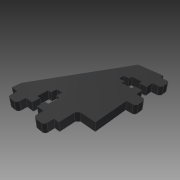
# Autodesk Inventor part: x_motor_cable_mount_brace
Saved by Autodesk Inventor 2014 (Build 180170000, 170)
## iProperties
Created: 2013-12-02
Part Number: x_motor_cable_mount_brace
Material: Generic
Document SubType Name: Modeling
Designer: buben
Density: 1 g/cm^3
Appearance: Anodized - Dark Gray
Author: buben
Subject: Laser Cutted
Autodesk Inventor part; units mm, degrees
ref_plane "YZ Plane" through (0, 0, 0) normal (1, 0, 0) x (0, 1, 0)
ref_plane "XZ Plane" through (0, 0, 0) normal (0, 1, 0) x (-1, 0, 0)
ref_plane "XY Plane" through (0, 0, 0) normal (0, 0, 1) x (1, 0, 0)
sketch "Sketch1" plane through (0, 0, 0) normal (0, 0, 1) x (1, 0, 0)
  line L0 (0, 0) -> (52, 0)
  line L1 (52, 0) -> (52, 68.9)
  line L2 (52, 68.9) -> (34, 68.9)
  line L3 (34, 68.9) -> (0, 6)
  line L4 (0, 6) -> (0, 0)
  dimension "d0" = 52
  dimension "d1" = 6
  dimension "d2" = 18
  dimension "d3" = 68.9
  constraints: 10 end point, 2 parallel, 1 horizontal, 1 perpendicular
  measures "d0" distance of L0.start L0.end
  measures "d1" distance of L3.end L0.start
  measures "d2" distance of L1.end L2.end
  measures "d3" distance of L0.end L1.end
extrude "Extrusion1" add sketch "Sketch1" along normal blind 6
sketch "Sketch2" plane through (0, 0, 6) normal (0, 0, 1) x (1, 0, 0)
  line L0 (0, 0) -> (52, 0) projected
  line L1 (52, 0) -> (52, 68.9) projected
  line L2 (18.75, 16.3) -> (23.25, 16.3)
  line L3 (23.25, 0) -> (18.75, 0)
  line L4 (25.75, 12.3) -> (25.75, 5)
  line L5 (16.25, 5) -> (16.25, 12.3)
  line L6 (39.7, 55.15) -> (47, 55.15)
  line L7 (47, 45.65) -> (39.7, 45.65)
  line L8 (52, 52.65) -> (52, 48.15)
  line L9 (35.7, 48.15) -> (35.7, 52.65)
  line L10 (16.25, 12.3) -> (18.75, 12.3)
  line L11 (23.25, 12.3) -> (25.75, 12.3)
  line L12 (18.75, 0) -> (18.75, 5)
  line L13 (18.75, 12.3) -> (18.75, 16.3)
  line L14 (25.75, 5) -> (23.25, 5)
  line L15 (18.75, 5) -> (16.25, 5)
  line L16 (23.25, 16.3) -> (23.25, 12.3)
  line L17 (23.25, 5) -> (23.25, 0)
  line L18 (52, 48.15) -> (47, 48.15)
  line L19 (39.7, 48.15) -> (35.7, 48.15)
  line L20 (35.7, 52.65) -> (39.7, 52.65)
  line L21 (47, 52.65) -> (52, 52.65)
  line L22 (39.7, 45.65) -> (39.7, 48.15)
  line L23 (39.7, 52.65) -> (39.7, 55.15)
  line L24 (47, 55.15) -> (47, 52.65)
  line L25 (47, 48.15) -> (47, 45.65)
  point P0 (35.7, 50.4)
  point P1 (21, 16.3)
  dimension "d6" = 4.5
  dimension "d7" = 2.5
  dimension "d8" = 2.5
  dimension "d9" = 5
  dimension "d10" = 4
  dimension "d11" = 7.3
  dimension "d12" = 4.5
  dimension "d13" = 2.5
  dimension "d14" = 2.5
  dimension "d15" = 4
  dimension "d16" = 5
  dimension "d17" = 7.3
  dimension "d19" = 31
  dimension "d39" = 18.5
  constraints: 48 end point, 20 parallel, 10 collinear, 8 perpendicular, 6 horizontal, 2 midpoint
  measures "d6" distance of L2.start L2.end
  measures "d7" distance of L11.start L4.start
  measures "d8" distance of L5.end L10.end
  measures "d9" distance of L14.end L3.start
  measures "d10" distance of L2.end L11.start
  measures "d11" distance of L4.start L4.end
  measures "d12" distance of L9.start L9.end
  measures "d13" distance of L20.end L6.start
  measures "d14" distance of L7.end L19.start
  measures "d15" distance of L19.start L9.start
  measures "d16" distance of L8.end L18.end
  measures "d17" distance of L7.start L7.end
  measures "d19" distance from line of L1 point (21, 16.3)
  measures "d39" vertical distance of L1.end point (35.7, 50.4)
extrude "Extrusion2" cut sketch "Sketch2" against normal blind 6
sketch "Sketch3" plane through (0, 0, 6) normal (0, 0, 1) x (1, 0, 0)
  line L0 (23.25, 0) -> (52, 0) projected
  line L1 (52, 0) -> (52, 48.15) projected
  line L2 (35.7, 48.15) -> (35.7, 52.65) projected
  line L3 (52, 52.65) -> (52, 68.9) projected
  line L4 (0, 0) -> (18.75, 0) projected
  line L5 (18.75, 16.3) -> (23.25, 16.3) projected
  line L6 (5.5, 0) -> (13.5, 0)
  line L7 (13.5, 0) -> (13.5, -4)
  line L8 (11.5, -6) -> (7.5, -6)
  line L9 (5.5, -4) -> (5.5, 0)
  line L10 (28.5, 0) -> (36.5, 0)
  line L11 (36.5, 0) -> (36.5, -4)
  line L12 (34.5, -6) -> (30.5, -6)
  line L13 (28.5, -4) -> (28.5, 0)
  line L14 (52, 34.9) -> (56, 34.9)
  line L15 (58, 36.9) -> (58, 40.9)
  line L16 (56, 42.9) -> (52, 42.9)
  line L17 (52, 42.9) -> (52, 34.9)
  line L18 (52, 65.9) -> (56, 65.9)
  line L19 (58, 63.9) -> (58, 59.9)
  line L20 (56, 57.9) -> (52, 57.9)
  line L21 (52, 57.9) -> (52, 65.9)
  arc A0 (5.5, -4) -> (7.5, -6) centre (7.5, -4) ccw
  arc A1 (11.5, -6) -> (13.5, -4) centre (11.5, -4) ccw
  arc A2 (28.5, -4) -> (30.5, -6) centre (30.5, -4) ccw
  arc A3 (34.5, -6) -> (36.5, -4) centre (34.5, -4) ccw
  arc A4 (56, 34.9) -> (58, 36.9) centre (56, 36.9) ccw
  arc A5 (58, 40.9) -> (56, 42.9) centre (56, 40.9) ccw
  arc A6 (58, 63.9) -> (56, 65.9) centre (56, 63.9) ccw
  arc A7 (56, 57.9) -> (58, 59.9) centre (56, 59.9) ccw
  point P0 (35.7, 50.4)
  point P1 (21, 16.3)
  dimension "d22" = 2
  dimension "d23" = 6
  dimension "d24" = 8
  dimension "d25" = 8
  dimension "d26" = 8
  dimension "d27" = 8
  dimension "d28" = 6
  dimension "d29" = 7.5
  dimension "d30" = 15
  dimension "d31" = 15
  dimension "d32" = 7.5
  constraints: 32 end point, 16 point on circle, 16 tangent, 8 centre point, 8 parallel, 7 equal radius, 4 horizontal, 4 perpendicular, 4 point on line, 2 collinear, 2 midpoint
  measures "d22" radius of A0
  measures "d23" distance between parallel lines of L3 L19
  measures "d24" distance between parallel lines of L20 L18
  measures "d25" distance between parallel lines of L14 L16
  measures "d26" distance between parallel lines of L7 L9
  measures "d27" distance between parallel lines of L11 L13
  measures "d28" distance between parallel lines of L4 L8
  measures "d29" distance from line of point (21, 16.3) L7
  measures "d30" distance between parallel lines of L13 L7
  measures "d31" distance between parallel lines of L16 L20
  measures "d32" distance from line of point (35.7, 50.4) L16
extrude "Extrusion3" add sketch "Sketch3" against normal blind 6
sketch "Sketch4" plane through (0, 0, 6) normal (0, 0, 1) x (1, 0, 0)
  line L0 (52, 0) -> (40, 0)
  line L1 (40, 0) -> (40, 12)
  line L2 (40, 12) -> (52, 12)
  line L3 (52, 12) -> (52, 0)
  dimension "d35" = 12
  dimension "d36" = 12
  constraints: 8 end point, 2 parallel, 1 horizontal, 1 perpendicular
  measures "d35" distance of L1.end L2.end
  measures "d36" distance of L0.end L1.end
extrude "Extrusion4" cut sketch "Sketch4" against normal blind 6
chamfer "Chamfer1" distance 2 angle 45 1 edges at (40, 12, 3)
body "Solid1"
